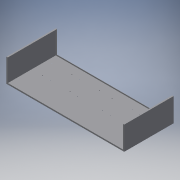
# Autodesk Inventor part: Ra-Manager_Base
Saved by Autodesk Inventor 2019.4 (Build 234330000, 330)
## iProperties
Created: 2020-03-10
Part Number: Ra-Manager_Base
Material: Genérico
Document SubType Name: Modeling
Designer: caio.santos
Density: 1 g/cm^3
Appearance: Padrão
Author: caio.santos
Autodesk Inventor part; units mm, degrees
ref_plane "YZ Plane" through (0, 0, 0) normal (1, 0, 0) x (0, 1, 0)
ref_plane "XZ Plane" through (0, 0, 0) normal (0, 1, 0) x (-1, 0, 0)
ref_plane "XY Plane" through (0, 0, 0) normal (0, 0, 1) x (1, 0, 0)
sketch "Esboço9" plane through (0, 0, 0) normal (0, 0, 1) x (1, 0, 0)
  line L0 (-215, -43.375) -> (215, -43.375)
  line L1 (215, -43.375) -> (215, 42.625)
  line L2 (215, 42.625) -> (214.25, 42.625)
  line L3 (214.25, 42.625) -> (214.25, -42.625)
  line L4 (214.25, -42.625) -> (-214.25, -42.625)
  line L5 (-214.25, -42.625) -> (-214.25, 42.625)
  line L6 (-214.25, 42.625) -> (-215, 42.625)
  line L7 (-215, 42.625) -> (-215, -43.375)
  point P0 (0, 0)
  dimension "d60" = 430
  dimension "d61" = 86
  dimension "d64" = 85.25
  dimension "d65" = 428.5
  dimension "d67" = 0.75
  dimension "d107" = 214.25
  dimension "d109" = 42.625
  constraints: 16 end point, 3 perpendicular, 2 horizontal, 2 point on line, 1 collinear, 1 parallel
  measures "d60" distance of L0.start L0.end
  measures "d61" distance of L0.end L1.end
  measures "d64" distance of L2.end L3.end
  measures "d65" distance of L3.end L4.end
  measures "d67" distance of L5.end L6.end
  measures "d107" distance from line of L5 point (0, 0)
  measures "d109" distance from line of point (0, 0) L4
extrude "Extrusão6" add sketch "Esboço9" against normal blind 180
sketch "Esboço10" plane through (-214.25, -42.625, 0) normal (0, 1, 0) x (1, 0, 0)
  line L0 (428.5, 0) -> (0, 0) projected
  line L1 (428.5, 0) -> (428.5, 0.75)
  line L2 (428.5, 0) -> (428.5, 180) projected
  line L3 (428.5, 0.75) -> (0, 0.75)
  line L4 (0, 0) -> (0, 180) projected
  line L5 (0, 180) -> (428.5, 180) projected
  line L6 (0, 180) -> (0, 179.25)
  line L7 (0, 0) -> (0, 180) projected
  line L8 (0, 179.25) -> (428.5, 179.25)
  line L9 (428.5, 179.25) -> (428.5, 180)
  line L10 (429.25, 180) -> (-0.75, 180) projected
  line L11 (0, 0.75) -> (0, 0)
  line L12 (-0.75, 0) -> (429.25, 0) projected
  line L13 (0, 180) -> (428.5, 180)
  point P0 (214.25, 0)
  dimension "d95" = 0.75
  dimension "d96" = 0.75
  constraints: 14 end point, 6 point on line, 3 perpendicular, 1 collinear
  measures "d95" distance of L0.start L1.end
  measures "d96" distance of L4.end L6.end
extrude "Extrusão7" add sketch "Esboço10" along normal blind 4.25 contours L0 L4 L3 L1 | L8 L4 L5 L2
sketch "Esboço11" plane through (214.25, 42.625, -180) normal (-1, 0, 0) x (0, 0, 1)
  line L0 (0, -81) -> (0.75, -81) projected
  line L1 (0.75, -81) -> (0, -81)
  line L2 (180, 0) -> (0, 0) projected
  line L3 (0, -81) -> (0, 0)
  line L4 (180, 0) -> (180, -81) projected
  line L5 (0, 0) -> (180, 0)
  line L6 (180, 0) -> (180, -81)
  line L7 (179.25, -81) -> (180, -81) projected
  line L8 (180, -81) -> (179.25, -81)
  line L9 (179.25, -81) -> (179.25, -0.75)
  line L10 (179.25, -0.75) -> (0.75, -0.75)
  line L11 (0.75, -0.75) -> (0.75, -81)
  point P0 (180, -42.625)
  dimension "d100" = 178.5
  dimension "d110" = 81
  dimension "d111" = 80.25
  constraints: 16 end point, 3 perpendicular, 2 collinear
  measures "d100" distance of L9.end L10.end
  measures "d110" distance of L2.start L4.end
  measures "d111" distance of L7.start L9.end
extrude "Extrusão8" add sketch "Esboço11" along normal blind 4.25
sketch "Esboço12" plane through (-214.25, 42.625, 0) normal (1, 0, 0) x (0, 0, -1)
  line L0 (0, -81) -> (0.75, -81) projected
  line L1 (0.75, -81) -> (0, -81)
  line L2 (0, -81) -> (0, 0)
  line L3 (180, -86) -> (180, 0) projected
  line L4 (0, 0) -> (180, 0)
  line L5 (179.25, -81) -> (180, -81) projected
  line L6 (180, 0) -> (180, -81)
  line L7 (180, -81) -> (179.25, -81)
  line L8 (179.25, -81) -> (179.25, -0.75)
  line L9 (179.25, -0.75) -> (0.75, -0.75)
  line L10 (0, -81) -> (0, 0) projected
  line L11 (0.75, -0.75) -> (0.75, -81)
  point P0 (0, -42.625)
  dimension "d103" = 80.25
  dimension "d104" = 178.5
  dimension "d112" = 81
  constraints: 16 end point, 4 perpendicular, 2 collinear
  measures "d103" distance of L5.start L8.end
  measures "d104" distance of L8.end L9.end
  measures "d112" distance of L3.end L5.end
extrude "Extrusão9" add sketch "Esboço12" along normal blind 4.25
sketch "Esboço15" plane through (-214.25, -42.625, -0.75) normal (0, 1, 0) x (1, 0, 0)
  circle A0 centre (311.2625, 145.825) radius 1.75 projected
  circle A1 centre (288.7625, 89.075) radius 1.75 projected
  line L0 (0, 0) -> (428.5, 0) projected
  line L1 (428.5, 0) -> (428.5, 178.5) projected
  line L2 (428.5, 178.5) -> (0, 178.5) projected
  line L3 (0, 0) -> (0, 178.5) projected
  circle A2 centre (260.7625, 89.075) radius 1.75 projected
  circle A3 centre (238.2625, 145.825) radius 1.75 projected
  circle A4 centre (192.2625, 145.825) radius 1.75 projected
  circle A5 centre (169.7625, 89.075) radius 1.75 projected
  circle A6 centre (141.7625, 89.075) radius 1.75 projected
  circle A7 centre (119.2625, 145.825) radius 1.75 projected
  circle A8 centre (91.2625, 145.825) radius 1.75 projected
  circle A9 centre (68.7625, 89.075) radius 1.75 projected
  circle A10 centre (40.7625, 89.075) radius 1.75 projected
  circle A11 centre (18.2625, 145.825) radius 1.75 projected
  circle A12 centre (339.2625, 145.825) radius 1.75 projected
  circle A13 centre (389.7875, 89.3) radius 1.75 projected
  circle A14 centre (412.2625, 145.825) radius 1.75 projected
  circle A15 centre (361.7875, 89.3) radius 1.75 projected
  point P0 (214.25, -0.75)
hole "Furo5" at (-195.9875, -42.625, -146.575) at (-122.9875, -42.625, -146.575) at (-145.4875, -42.625, -89.825) at (-173.4875, -42.625, -89.825) at (-94.9875, -42.625, -146.575) at (-72.4875, -42.625, -89.825) at (-44.4875, -42.625, -89.825) at (-21.9875, -42.625, -146.575) at (24.0125, -42.625, -146.575) at (46.5125, -42.625, -89.825) at (74.5125, -42.625, -89.825) at (97.0125, -42.625, -146.575) at (125.0125, -42.625, -146.575) at (198.0125, -42.625, -146.575) at (175.5375, -42.625, -90.05) at (147.5375, -42.625, -90.05) direction (0, -1, 0) diameter 2.459 end through all thread size "M3x0.5" class "6H" standard "ANSI Metric M Profile"
equation "\"d107\" = 0.5 * d65"
equation "\"d109\" = 0.5 * d64"
